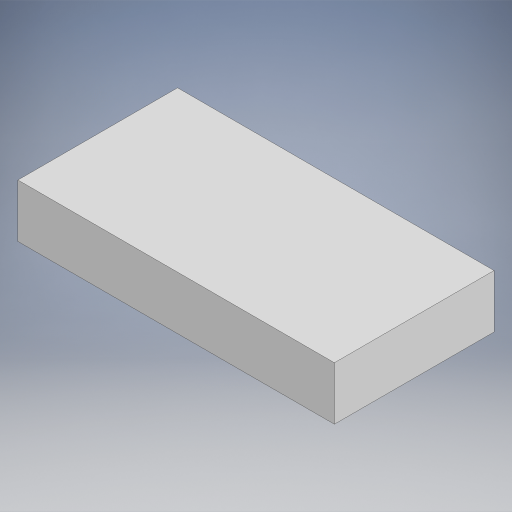
# Autodesk Inventor part: Part3
Saved by Autodesk Inventor 2023 (Build 270158000, 158)
## iProperties
Created: 2022-10-20
Part Number: Part3
Material: Generic
Document SubType Name: Modeling
Designer: awelt
Mass: 63137.7 g
Surface Area: 12441.3 cm^2
Volume: 63137.7 cm^3
Density: 1 g/cm^3
Appearance: Default
RuleStatus: InUse
AfterAnyParamChange0: BoundingBox
AfterAnyiPropertyChange0: BoundingBox
PartBodyChanged0: BoundingBox
Author: awelt
BoundingBL1: 6
BoundingBL2: 18
BoundingBL3: 35 11/16
BoundingCF: 2.23
Autodesk Inventor part; units mm, degrees
ref_plane "YZ Plane" through (0, 0, 0) normal (1, 0, 0) x (0, 1, 0)
ref_plane "XZ Plane" through (0, 0, 0) normal (0, 1, 0) x (-1, 0, 0)
ref_plane "XY Plane" through (0, 0, 0) normal (0, 0, 1) x (1, 0, 0)
sketch "Sketch2" plane through (0, 0, 0) normal (1, 0, 0) x (0, 1, 0)
  line L0 (0.2037, 0) -> (152.6037, 0)
  line L1 (152.6037, 0) -> (152.6037, -457.2)
  line L2 (152.6037, -457.2) -> (0.2037, -457.2)
  line L3 (0.2037, -457.2) -> (0.2037, 0)
  point P0 (0, 0)
  dimension "d4" = 152.4
  dimension "d5" = 457.2
  constraints: 8 end point, 2 parallel, 1 horizontal, 1 perpendicular
  measures "d4" distance of L1.end L2.end
  measures "d5" distance of L0.end L1.end
extrude "Extrusion2" add sketch "Sketch2" along normal blind 906.145
body "Solid2"
